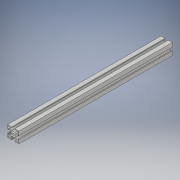
# Autodesk Inventor part: extrusion_300
Saved by Autodesk Inventor 2019.3 (Build 233278000, 278)
## iProperties
Created: 2019-04-14
Part Number: extrusion_300
Material: Generic
Document SubType Name: Modeling
Designer: peter
Density: 1 g/cm^3
Appearance: Default
Author: peter
Autodesk Inventor part; units mm, degrees
ref_plane "YZ Plane" through (0, 0, 0) normal (1, 0, 0) x (0, 1, 0)
ref_plane "XZ Plane" through (0, 0, 0) normal (0, 1, 0) x (-1, 0, 0)
ref_plane "XY Plane" through (0, 0, 0) normal (0, 0, 1) x (1, 0, 0)
sketch "Sketch1" plane through (0, 0, 0) normal (0, 0, 1) x (1, 0, 0)
  line L0 (0, 0) -> (8, 0)
  line L1 (8, 0) -> (8, -1.5)
  line L2 (8, -1.5) -> (5.5711, -1.5)
  line L3 (0, -1.5) -> (0, 0)
  line L4 (0, 0) -> (5, 0) construction
  line L5 (4.2426, -2.8284) -> (5.5711, -1.5)
  line L6 (6.5, -14.0858) -> (6.5, -7.9142)
  line L7 (7.9142, -6.5) -> (15.5, -6.5)
  line L8 (0, -8) -> (1.5, -8)
  line L9 (1.5, -8) -> (1.5, -5.5711)
  line L10 (11, -11) -> (10.2929, -10.2929) construction
  line L11 (11, -11) -> (10.2929, -11.7071) construction
  line L12 (0, 0) -> (8, 0)
  line L13 (5.5711, -1.5) -> (4.2426, -2.8284)
  line L14 (2.8284, -4.2426) -> (1.5, -5.5711)
  line L15 (7.9142, -6.5) -> (4.2426, -2.8284)
  line L16 (6.5, -7.9142) -> (2.8284, -4.2426)
  circle A0 centre (11, -11) radius 2
  line L17 (11, -11) -> (16.6687, -11) construction
  line L18 (11, -16.9105) -> (11, -11) construction
  line L19 (22, 0) -> (14, 0)
  line L20 (14, 0) -> (14, -1.5)
  line L21 (14, -1.5) -> (16.4289, -1.5)
  line L22 (22, -1.5) -> (22, 0)
  line L23 (22, 0) -> (17, 0)
  line L24 (17.7574, -2.8284) -> (16.4289, -1.5)
  line L25 (15.5, -15.5) -> (15.5, -7.9142)
  line L26 (15.5, -6.5) -> (7.9142, -6.5)
  line L27 (22, -8) -> (20.5, -8)
  line L28 (20.5, -8) -> (20.5, -5.5711)
  line L29 (11, -11) -> (11.7071, -10.2929) construction
  line L30 (11, -11) -> (11.7071, -11.7071) construction
  line L31 (22, 0) -> (14, 0)
  line L32 (16.4289, -1.5) -> (17.7574, -2.8284)
  line L33 (19.1716, -4.2426) -> (20.5, -5.5711)
  line L34 (14.0858, -6.5) -> (17.7574, -2.8284)
  line L35 (15.5, -7.9142) -> (19.1716, -4.2426)
  circle A1 centre (11, -11) radius 2
  line L36 (0, -22) -> (8, -22)
  line L37 (8, -22) -> (8, -20.5)
  line L38 (8, -20.5) -> (5.5711, -20.5)
  line L39 (0, -20.5) -> (0, -22)
  line L40 (0, -22) -> (5, -22) construction
  line L41 (4.2426, -19.1716) -> (5.5711, -20.5)
  line L42 (6.5, -7.9142) -> (6.5, -14.0858)
  line L43 (6.5, -15.5) -> (14.0858, -15.5)
  line L44 (0, -14) -> (1.5, -14)
  line L45 (1.5, -14) -> (1.5, -16.4289)
  line L46 (11, -11) -> (10.2929, -11.7071) construction
  line L47 (11, -11) -> (10.2929, -10.2929) construction
  line L48 (0, -22) -> (8, -22)
  line L49 (5.5711, -20.5) -> (4.2426, -19.1716)
  line L50 (2.8284, -17.7574) -> (1.5, -16.4289)
  line L51 (7.9142, -15.5) -> (4.2426, -19.1716)
  line L52 (6.5, -14.0858) -> (2.8284, -17.7574)
  circle A2 centre (11, -11) radius 2
  line L53 (22, -22) -> (14, -22)
  line L54 (14, -22) -> (14, -20.5)
  line L55 (14, -20.5) -> (16.4289, -20.5)
  line L56 (22, -20.5) -> (22, -22)
  line L57 (22, -22) -> (17, -22)
  line L58 (17.7574, -19.1716) -> (16.4289, -20.5)
  line L59 (20.5, -14) -> (20.5, -16.4289)
  line L60 (15.5, -14.0858) -> (19.1716, -17.7574)
  line L61 (19.1716, -17.7574) -> (20.5, -16.4289)
  line L62 (14.0858, -15.5) -> (17.7574, -19.1716)
  line L63 (16.4289, -20.5) -> (17.7574, -19.1716)
  line L64 (22, -22) -> (14, -22)
  line L65 (22, -14) -> (20.5, -14)
  line L66 (11, -11) -> (11.7071, -11.7071) construction
  line L67 (11, -11) -> (11.7071, -10.2929) construction
  line L68 (14.0858, -15.5) -> (6.5, -15.5)
  line L69 (15.5, -7.9142) -> (15.5, -15.5)
  circle A3 centre (11, -11) radius 2
  line L70 (22, -14) -> (22, -20.5)
  line L71 (22, -1.5) -> (22, -8)
  line L72 (8, 0) -> (0, 0) construction
  line L73 (0, 0) -> (0, -8) construction
  line L74 (9.5858, -11) -> (9.0681, -11.5176)
  line L75 (6.5, -14.0858) -> (2.8284, -17.7574)
  line L76 (0, -22) -> (0, -14)
  line L77 (0, -8) -> (0, 0)
  line L78 (0, 0) -> (2, 0) construction
  line L79 (2, 0) -> (2, -2) construction
  circle A4 centre (2, -2) radius 1
  circle A5 centre (20, -2) radius 1
  circle A6 centre (2, -20) radius 1
  circle A7 centre (20, -20) radius 1
  point P0 (3.5355, -3.5355)
  point P1 (0, -7.0711)
  point P2 (6.5, -6.5)
  point P3 (6.5, -15.5)
  point P4 (1.5, 0)
  point P5 (10.2929, -10.2929)
  point P6 (18.4645, -3.5355)
  point P7 (22, -7.0711)
  point P8 (6.5, -6.5)
  point P9 (20.5, 0)
  point P10 (11.7071, -10.2929)
  point P11 (12.4142, -11)
  point P12 (3.5355, -18.4645)
  point P13 (0, -14.9289)
  point P14 (6.5, -6.5)
  point P15 (1.5, -22)
  point P16 (10.2929, -11.7071)
  point P17 (18.4645, -18.4645)
  point P18 (20.5, -22)
  point P19 (22, -14.9289)
  point P20 (15.5, -6.5)
  point P21 (11.7071, -11.7071)
  dimension "d2" = 8
  dimension "d3" = 1.5
  dimension "d4" = 5
  dimension "d10" = 9
  dimension "d11" = 9
  dimension "d14" = 4
  dimension "d15" = 2
  dimension "d16" = 2
  dimension "d17" = 2
  constraints: 160 end point, 68 symmetric about line, 7 centre point, 5 coincident, 5 point on line, 4 collinear, 4 horizontal, 3 perpendicular, 2 parallel, 1 line through centre, 1 vertical, 8 other
  measures "d2" distance of L1.end L3.start
  measures "d3" distance of L0.end L1.end
  measures "d4" distance of L0.start point (3.536, -3.536)
  measures "d10" distance of point (6.5, -6.5) L7.end
  measures "d11" distance of point (6.5, -15.5) point (6.5, -6.5)
  measures "d14" diameter of A0
  measures "d15" distance of L0.start L78.end
  measures "d16" distance of L78.end L79.end
  measures "d17" diameter of A4
extrude "Extrusion1" add sketch "Sketch1" along normal blind 300
body "Solid1"
